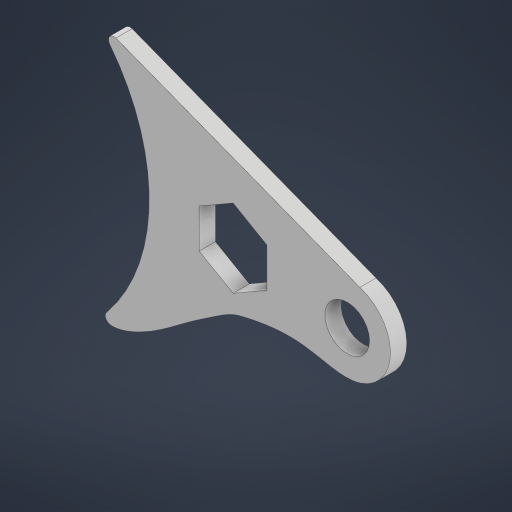
# Autodesk Inventor part: gear-interface
Saved by Autodesk Inventor 2023.2 (Build 272271000, 271)
## iProperties
Created: 2023-03-20
Part Number: gear-interface
Material: Generic
Document SubType Name: Modeling
Designer: Liam
Density: 1 g/cm^3
Appearance: Default
Author: Liam
Autodesk Inventor part; units mm, degrees
ref_plane "YZ Plane" through (0, 0, 0) normal (1, 0, 0) x (0, 1, 0)
ref_plane "XZ Plane" through (0, 0, 0) normal (0, 1, 0) x (-1, 0, 0)
ref_plane "XY Plane" through (0, 0, 0) normal (0, 0, 1) x (1, 0, 0)
sketch "Sketch1" plane through (0, 0, 0) normal (0, 0, 1) x (1, 0, 0)
  line L0 (25.3998, 3.6661) -> (28.5748, 1.833)
  line L1 (28.5748, -1.8332) -> (28.5748, 1.833)
  line L2 (28.5748, -1.8332) -> (25.3998, -3.6663)
  line L3 (22.2248, -1.8332) -> (25.3998, -3.6663)
  line L4 (22.2248, -1.8332) -> (22.2248, 1.833)
  line L5 (25.3998, 3.6661) -> (22.2248, 1.833)
  line L6 (37.2896, 2.7532) -> (14.4086, 11.5688)
  arc A0 (14.4086, 11.5688) -> (13.8254, 10.7824) centre (14.226, 11.0948) ccw
  arc A1 (13.5904, -11.0771) -> (13.663, -11.9077) centre (13.9159, -11.4671) ccw
  arc A2 (37.3783, -4.9776) -> (37.2896, 2.7532) centre (36.1099, -1.1262) ccw
  arc A3 (13.5904, -11.0771) -> (13.8254, 10.7824) centre (0, 0) ccw
  circle A4 centre (36.1099, -1.1262) radius 2.0955
  line L7 (13.663, -11.9077) -> (14.2788, -12.2612) construction
  line L8 (14.2788, -12.2612) -> (17.5318, -11.0771) construction
  line L9 (17.5318, -11.0771) -> (20.5276, -8.439) construction
  line L10 (20.5276, -8.439) -> (23.3977, -6.6512) construction
  line L11 (23.3977, -6.6512) -> (25.2547, -5.247) construction
  line L12 (25.2547, -5.247) -> (26.8437, -5.0222) construction
  line L13 (26.8437, -5.0222) -> (28.4342, -4.5899) construction
  line L14 (28.4342, -4.5899) -> (32.6217, -4.2251) construction
  line L15 (32.6217, -4.2251) -> (35.64, -5.5501) construction
  line L16 (35.64, -5.5501) -> (37.3783, -4.9776) construction
  spline S0 degree 4 poles (13.663, -11.9077) (14.2788, -12.2612) (17.5318, -11.0771) (20.5276, -8.439) (23.3977, -6.6512) (25.2547, -5.247) (26.8437, -5.0222) (28.4342, -4.5899) (32.6217, -4.2251) (35.64, -5.5501) (37.3783, -4.9776) knots 1 1 1 1 1 2 3 4 5 6 7 8 8 8 8 8
  point P0 (0, 0)
  point P1 (16.4691, 5.9941)
  point P2 (16.469, -5.9943)
  point P3 (25.3998, -0.0001)
  dimension "d31" = 3.6662
  dimension "d32" = 3.6662
  dimension "d34" = 3.6662
  dimension "d35" = 3.6662
  dimension "d36" = 3.6662
  dimension "d37" = 3.6662
  dimension "d39" = 4.191
  constraints: 14 end point, 8 point on circle, 5 centre point, 5 equal length, 2 tangent, 1 coincident, 1 equal radius, 1 vertical, 11 other
  measures "d31" distance of point (25.4, 0) L4.end
  measures "d32" distance of L0.start point (25.4, 0)
  measures "d34" distance of L0.end point (25.4, 0)
  measures "d35" distance of L1.start point (25.4, 0)
  measures "d36" distance of L2.end point (25.4, 0)
  measures "d37" distance of point (25.4, 0) L3.start
  measures "d39" diameter of A4
extrude "Extrusion6" add sketch "Sketch1" along normal blind 1.524
equation "\"d32\" = d31"
equation "\"d34\" = d31"
equation "\"d35\" = d31"
equation "\"d36\" = d31"
equation "\"d37\" = d31"
body "Solid6"
